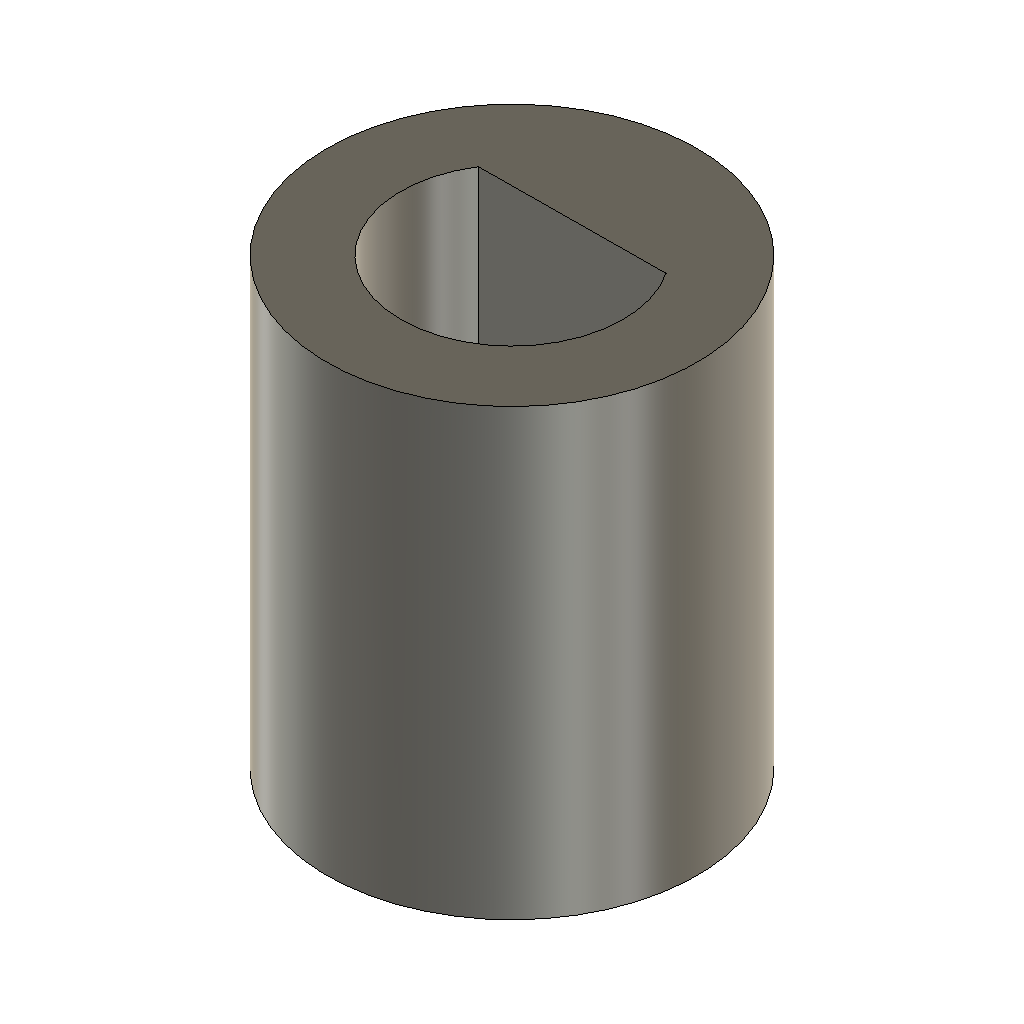
3mm too 5mm shaft (Autodesk Fusion 360 design; units mm, degrees)
part number: 2026-09-19-16-53-31-621
Autodesk Fusion 360 part; units mm, degrees
note: some values were not read from the file. Set by a fixed rule: which sketch regions a step uses.
sketch "Sketch1" plane through (0, 0, 0) normal (0, 0, 1) x (1, 0, 0)
  circle A0 centre (0, 0) radius 2.5
  dimension "d1" = 5
  constraint coincident A0.centre origin
  measures "d1" diameter of A0
extrude "Extrude1" add sketch "Sketch1" along normal blind 6
sketch "Sketch2" plane through (0, 0, 6) normal (0, 0, 1) x (-1, 0, 0)
  circle A0 centre (0, 0) radius 2.5
  circle A1 centre (0, 0) radius 1.5
  dimension "d4" = 3
  constraint concentric A0 A1
  measures "d4" diameter of A1
extrude "Extrude2" cut sketch "Sketch2" against normal blind 5 contours A1
sketch "Sketch3" plane through (0, 0, 1) normal (0, 0, 1) x (-1, 0, 0)
  circle A0 centre (0, 0) radius 1.5
  line L0 (1.2625, -0.8099) -> (-1.2492, -0.8303)
  arc A1 (0.0066, -1.5) -> (-1.2492, -0.8303) centre (0, 0) ccw
  constraint coincident A0 L0.start
  constraint coincident A0 L0.end
  constraint coincident L0.start A1
  constraint coincident A0 A1.start
extrude "Extrude3" add sketch "Sketch3" along normal blind 5 contours A0 L0 A1 picked at (0.6944, -1.19)
